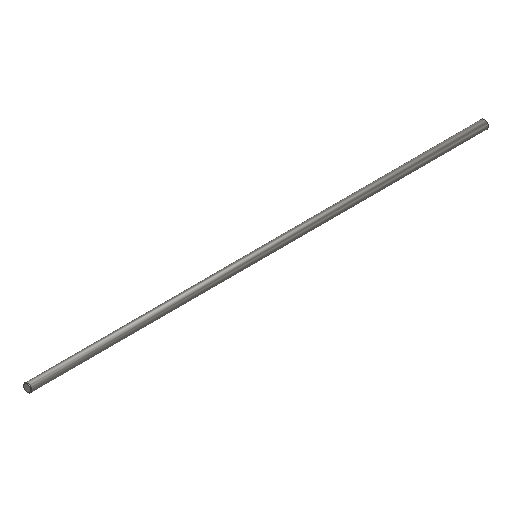
# Autodesk Inventor part: CUT_STEEL_8x434mm_Linear_rod
Saved by Autodesk Inventor 2026.1 (Build 301233000, 233)
## iProperties
Created: 2018-06-17
Part Number: CUT_STEEL_8x434mm_Linear_rod
Material: Stainless Steel
Document SubType Name: Modeling
Designer: Andrzej
Density: 8 g/cm^3
Appearance: Semi-Polished
Author: Andrzej
Autodesk Inventor part; units mm, degrees
ref_plane "YZ Plane" through (0, 0, 0) normal (1, 0, 0) x (0, 1, 0)
ref_plane "XZ Plane" through (0, 0, 0) normal (0, 1, 0) x (-1, 0, 0)
ref_plane "XY Plane" through (0, 0, 0) normal (0, 0, 1) x (1, 0, 0)
sketch "Sketch1" plane through (0, 0, 0) normal (0, 0, 1) x (1, 0, 0)
  circle A0 centre (0, 0) radius 4
  dimension "d0" = 8
  constraints: 1 centre point, 1 coincident
  measures "d0" diameter of A0
extrude "Extrusion1" add sketch "Sketch1" along normal blind 434
chamfer "Chamfer1" distance 0.5 angle 45 2 edges at (-4, 0, 434) (-4, 0, 0)
body "Solid1"
